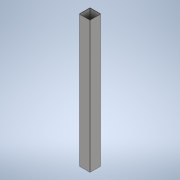
# Autodesk Inventor part: 21015-22-1-3- 6X6 Stanchion
Saved by Autodesk Inventor 2022 (Build 260153000, 153)
## iProperties
Created: 2021-06-17
Part Number: 21015-22-1-3- 6X6 Stanchion
Material: Steel, Carbon
Document SubType Name: Modeling
Designer: Skynet
Density: 7.85 g/cm^3
Appearance: Semi-Polished
Mass: 40014.2 g
Surface Area: 21405 cm^2
Volume: 5097.35 cm^3
Author: Skynet
Autodesk Inventor part; units mm, degrees
ref_plane "YZ Plane" through (0, 0, 0) normal (1, 0, 0) x (0, 1, 0)
ref_plane "XZ Plane" through (0, 0, 0) normal (0, 1, 0) x (-1, 0, 0)
ref_plane "XY Plane" through (0, 0, 0) normal (0, 0, 1) x (1, 0, 0)
sketch "Sketch1" plane through (0, 0, 0) normal (0, 1, 0) x (-1, 0, 0)
  line L0 (6.35, 0) -> (146.05, 0)
  line L1 (152.4, -6.35) -> (152.4, -146.05)
  line L2 (146.05, -152.4) -> (6.35, -152.4)
  line L3 (0, -146.05) -> (0, -6.35)
  arc A0 (146.05, -152.4) -> (152.4, -146.05) centre (146.05, -146.05) ccw
  arc A1 (152.4, -6.35) -> (146.05, 0) centre (146.05, -6.35) ccw
  arc A2 (0, -146.05) -> (6.35, -152.4) centre (6.35, -146.05) ccw
  arc A3 (152.4, -6.35) -> (146.05, 0) centre (146.05, -6.35) ccw
  arc A4 (6.35, 0) -> (0, -6.35) centre (6.35, -6.35) ccw
  line L4 (147.6248, -146.05) -> (147.6248, -6.35)
  arc A5 (147.6248, -6.35) -> (146.05, -4.7752) centre (146.05, -6.35) ccw
  line L5 (146.05, -4.7752) -> (6.35, -4.7752)
  arc A6 (6.35, -4.7752) -> (4.7752, -6.35) centre (6.35, -6.35) ccw
  line L6 (4.7752, -6.35) -> (4.7752, -146.05)
  arc A7 (4.7752, -146.05) -> (6.35, -147.6248) centre (6.35, -146.05) ccw
  line L7 (6.35, -147.6248) -> (146.05, -147.6248)
  arc A8 (146.05, -147.6248) -> (147.6248, -146.05) centre (146.05, -146.05) ccw
  point P0 (0, 0)
  point P1 (152.4, -152.4)
  point P2 (152.4, 0)
  point P3 (0, -152.4)
  dimension "d0" = 152.4
  dimension "d1" = 152.4
  dimension "d2" = 6.35
  dimension "d3" = 6.35
  dimension "d4" = 6.35
  dimension "d5" = 4.7752
  constraints: 18 point on circle, 16 end point, 10 point on line, 10 tangent, 9 centre point, 4 parallel, 2 equal radius, 2 perpendicular, 1 horizontal, 7 other
  measures "d0" distance of point (152.4, 0) point (152.4, -152.4)
  measures "d1" distance of point (152.4, -152.4) point (0, -152.4)
  measures "d2" radius of A0
  measures "d3" radius of A3
  measures "d4" radius of A4
  measures "d5" distance between parallel lines of L1 L4
extrude "Extrusion1" add sketch "Sketch1" along normal blind 1828.8
body "Solid1"
